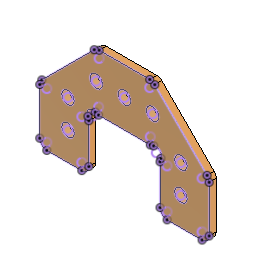
Custom Short U-Bracket (Autodesk Fusion 360 design; units mm, degrees)
Autodesk Fusion 360 part; units mm, degrees
sketch "Sketch1" plane through (0, 0, 0) normal (0, 1, 0) x (1, 0, 0)
  line L0 (0, 0) -> (0, -25.4)
  line L1 (76.2, -25.4) -> (76.2, 0)
  line L2 (76.2, 0) -> (54.102, 0)
  line L3 (54.102, 0) -> (54.102, -25.4)
  line L4 (54.102, -25.4) -> (22.098, -25.4)
  line L5 (22.098, -25.4) -> (22.098, 0)
  line L6 (22.098, 0) -> (0, 0)
  line L7 (38.1, -25.4) -> (38.1, -50.8) construction
  circle A0 centre (23.7818, -23.7162) radius 2.3813
  line L8 (23.7818, -23.7162) -> (23.7818, -25.4) construction
  line L9 (23.7818, -23.7162) -> (22.098, -23.7162) construction
  circle A1 centre (12.7, -12.7) radius 2.7781
  line L10 (0, -25.4) -> (25.4, -50.8)
  line L11 (25.4, -50.8) -> (50.8, -50.8)
  line L12 (50.8, -50.8) -> (76.2, -25.4)
  circle A2 centre (12.7, -25.4) radius 2.7781
  circle A3 centre (25.4, -38.1) radius 2.7781
  circle A4 centre (38.1, -38.1) radius 2.7781
  circle A5 centre (50.8, -38.1) radius 2.7781
  circle A6 centre (63.5, -12.7) radius 2.7781
  circle A7 centre (63.5, -25.4) radius 2.7781
  circle A8 centre (52.4182, -23.7162) radius 2.3813
  dimension "d1" = 76.2
  dimension "d3" = 32.004
  dimension "d4" = 25.4
  dimension "d6" = 25.4
  dimension "d8" = 4.7625
  dimension "d9" = 5.5563
  dimension "d10" = 12.7
  dimension "d26" = 25.4
  dimension "d43" = 25.4
  dimension "d44" = 12.7
  dimension "d47" = -25.4
  dimension "d48" = -50.8
  constraint coincident L0.start L6.end
  constraint vertical L0
  constraint perpendicular L1 L2
  constraint perpendicular L2 L3
  constraint perpendicular L3 L4
  constraint perpendicular L4 L5
  constraint perpendicular L0 L6
  constraint equal L2 L6
  constraint midpoint L4 L7.start
  constraint equal L0 L1
  constraint coincident L4.end A0
  constraint coincident A0.centre L8.start
  constraint coincident L4 L8.end
  constraint perpendicular L4 L8
  constraint coincident L5 L9.end
  constraint perpendicular L5 L9
  constraint equal L8 L9
  constraint perpendicular L0 L11
  constraint equal L10 L12
  constraint collinear L2 L6
  constraint coincident L7.end L11
  constraint symmetric L7 A0 A8
  constraint midpoint L7.end L11
  measures "d1" distance of L0 L1
  measures "d3" distance of L3.end L4.end
  measures "d4" distance of L4.end L5.end
  measures "d6" distance of L0.start L0.end
  measures "d8" diameter of A0
  measures "d9" diameter of A1
  measures "d10" distance of L6 A1.centre
  measures "d26" distance of L10.end L11.end
  measures "d43" distance of L4 L11
  measures "d44" distance of L0 A1.centre
extrude "Extrude1" add sketch "Sketch1" along normal blind 3.175 contours L0 L1 L2 L3 L4 L5 L6 A0 L10 L11 L12 A8
fillet "Fillet1" radius 3.175 8 edges at (0, 1.5875, 0) (22.098, 1.5875, 0) (54.102, 1.5875, 0) (76.2, 1.5875, 0) (0, 1.5875, 25.4) (25.4, 1.5875, 50.8) (50.8, 1.5875, 50.8) (76.2, 1.5875, 25.4)
fillet "Fillet1" radius 3.175 4 edges at (25.4656, 1.5875, 25.4) (22.098, 1.5875, 22.0324) (50.7344, 1.5875, 25.4) (54.102, 1.5875, 22.0324)
sketch "DXF" plane through (0, 0, 0) normal (0, -1, 0) x (1, 0, 0)
  circle A0 centre (38.1, 38.1) radius 2.7781
  circle A1 centre (12.7, 12.7) radius 2.7781
  circle A2 centre (25.4, 38.1) radius 2.7781
  circle A3 centre (12.7, 25.4) radius 2.7781
  circle A4 centre (63.5, 12.7) radius 2.7781
  circle A5 centre (63.5, 25.4) radius 2.7781
  circle A6 centre (50.8, 38.1) radius 2.7781
  arc A7 (54.5005, 22.5611) -> (54.102, 21.021) centre (57.277, 21.021) ccw
  line L0 (54.102, 21.021) -> (54.102, 3.175)
  arc A8 (54.102, 3.175) -> (57.277, 0) centre (57.277, 3.175) ccw
  line L1 (57.277, 0) -> (73.025, 0)
  arc A9 (73.025, 0) -> (76.2, 3.175) centre (73.025, 3.175) ccw
  line L2 (76.2, 3.175) -> (76.2, 24.0849)
  arc A10 (76.2, 24.0849) -> (75.2701, 26.3299) centre (73.025, 24.0849) ccw
  line L3 (75.2701, 26.3299) -> (51.7299, 49.8701)
  arc A11 (51.7299, 49.8701) -> (49.4849, 50.8) centre (49.4849, 47.625) ccw
  line L4 (49.4849, 50.8) -> (26.7151, 50.8)
  arc A12 (26.7151, 50.8) -> (24.4701, 49.8701) centre (26.7151, 47.625) ccw
  line L5 (24.4701, 49.8701) -> (0.9299, 26.3299)
  arc A13 (0.9299, 26.3299) -> (0, 24.0849) centre (3.175, 24.0849) ccw
  line L6 (0, 24.0849) -> (0, 3.175)
  arc A14 (0, 3.175) -> (3.175, 0) centre (3.175, 3.175) ccw
  line L7 (3.175, 0) -> (18.923, 0)
  arc A15 (18.923, 0) -> (22.098, 3.175) centre (18.923, 3.175) ccw
  line L8 (22.098, 3.175) -> (22.098, 21.021)
  arc A16 (22.098, 21.021) -> (21.6995, 22.5611) centre (18.923, 21.021) ccw
  arc A17 (24.9369, 25.7985) -> (21.6995, 22.5611) centre (23.7818, 23.7162) ccw
  arc A18 (24.9369, 25.7985) -> (26.477, 25.4) centre (26.477, 28.575) ccw
  line L9 (26.477, 25.4) -> (49.723, 25.4)
  arc A19 (49.723, 25.4) -> (51.2631, 25.7985) centre (49.723, 28.575) ccw
  arc A20 (54.5005, 22.5611) -> (51.2631, 25.7985) centre (52.4182, 23.7162) ccw
equation "TOLERANCE = 0.01 in" comment "Tube size tolerance"
equation "d3 = 1 in + 2 * PLATE_THICKNESS + TOLERANCE"
equation "d9 = ( 7 / 32 ) * 1 in"
equation "HOLE_DIAMETER = ( 7 / 32 ) * 1 in"
equation "PLATE_THICKNESS = 0.125 in" comment "Non-zero if you want this to overlap other plates"
